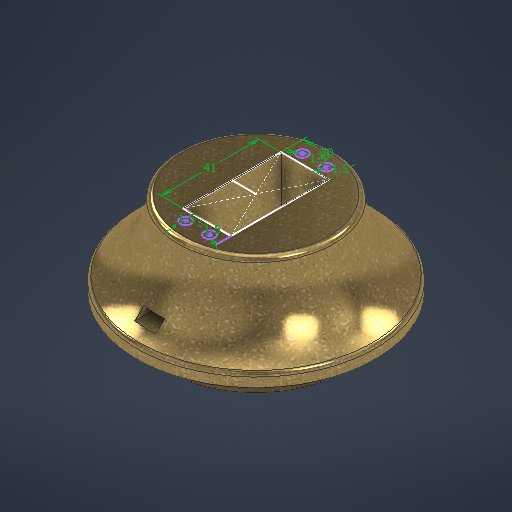
# Autodesk Inventor part: Pieza3
Saved by Autodesk Inventor 2026.1 (Build 301233020, 233B)
## iProperties
Created: 2026-05-16
Part Number: Pieza3
Material: Genérico
Document SubType Name: Modeling
Designer: USUARIO
Density: 1 g/cm^3
Appearance: Valor por defecto
Author: USUARIO
Autodesk Inventor part; units mm, degrees
ref_plane "YZ Plane" through (0, 0, 0) normal (1, 0, 0) x (0, 1, 0)
ref_plane "XZ Plane" through (0, 0, 0) normal (0, 1, 0) x (-1, 0, 0)
ref_plane "XY Plane" through (0, 0, 0) normal (0, 0, 1) x (1, 0, 0)
sketch "Boceto1" plane through (0, 0, 0) normal (1, 0, 0) x (0, 1, 0)
  line L0 (0, 0) -> (0, 32.5)
  line L1 (0, 0) -> (32.5, 0) construction
  line L2 (0, 0) -> (-35, 0)
  line L3 (0, 0) -> (35, 0) construction
  line L4 (-35, 0) -> (-35, 50)
  line L5 (-35, 0) -> (15, 0) construction
  line L6 (-35, 50) -> (-30, 50)
  line L7 (-35, 50) -> (-30, 50) construction
  arc A0 (-30, 50) -> (0, 32.5) centre (-0.3993, 66.2798) ccw
  dimension "d1" = 90
  dimension "d3" = 35
  dimension "d4" = 180
  dimension "d5" = 50
  dimension "d6" = 90
  dimension "d7" = 5
  dimension "d8" = 0
  constraints: 16 end point, 6 horizontal, 4 equal length, 2 point on circle, 2 vertical, 1 centre point
  measures "d1" angle of L1 L0
  measures "d3" distance of L0.start L2.end
  measures "d4" angle of L2 L3
  measures "d5" distance of L2.end L4.end
  measures "d6" angle of L5 L4
  measures "d7" distance of L4.end L6.end
  measures "d8" distance between parallel lines of L6 L7
revolve "Revolución1" add sketch "Boceto1" angle 360 about axis through (0, 0, 0) along (0, -1, 0)
fillet "Empalme1" radius 2 2 edges at (0, 0, -32.5) (0, -30, -50)
sketch "Boceto2" plane through (0, 0, 0) normal (0, 1, 0) x (1, 0, 0)
  line L0 (10, -20.5) -> (-10, -20.5)
  line L1 (-10, -20.5) -> (-10, 20.5)
  line L2 (-10, 20.5) -> (10, 20.5)
  line L3 (10, 20.5) -> (10, -20.5)
  line L4 (10, -20.5) -> (-10, 20.5) construction
  line L5 (-10, -20.5) -> (10, 20.5) construction
  line L6 (10, -20.5) -> (-10, -20.5)
  line L7 (10, -27) -> (10, -20.5)
  line L8 (10, -20.5) -> (-10, -20.5)
  line L9 (10, -23.5) -> (10, -20.5)
  line L10 (-10, -20.5) -> (-6, -20.5) construction
  circle A0 centre (-5, -24.5) radius 2.2
  circle A1 centre (5, -24.5) radius 2.2
  line L11 (0, 0) -> (-10, 0)
  circle A2 centre (-5, 24.5) radius 2.2
  circle A3 centre (5, 24.5) radius 2.2
  circle A4 centre (-5, 24.5) radius 0.75
  circle A5 centre (5, 24.5) radius 0.75
  circle A6 centre (-5, -24.5) radius 0.75
  circle A7 centre (5, -24.5) radius 0.75
  dimension "d11" = 20
  dimension "d12" = 41
  dimension "d34" = 1.5
  dimension "d35" = 1.5
  dimension "d36" = 1.5
  dimension "d37" = 1.5
  constraints: 24 end point, 8 centre point, 4 coincident, 4 horizontal, 3 midpoint, 2 parallel, 2 symmetric about line, 1 perpendicular, 2 other
  measures "d11" distance of L1.end L2.end
  measures "d12" distance of L0.end L1.end
  measures "d34" diameter of A4
  measures "d35" diameter of A5
  measures "d36" diameter of A6
  measures "d37" diameter of A7
extrude "Extrusión1" cut sketch "Boceto2" against normal blind 8 contours A0 | A1 | A2 | A3 | A4 | A5 | A6 | A7
extrude "Extrusión2" cut sketch "Boceto2" against normal blind 30 contours L0 L1 L2 L3
sketch "Boceto3" plane through (0, -35, 0) normal (0, -1, 0) x (1, 0, 0)
  circle A0 centre (0, 0) radius 38.5
  line L0 (38.5, 5) -> (5, 5)
  line L1 (-5, 5) -> (-38.5, 5)
  line L2 (5, 38.5) -> (5, 5)
  line L3 (5, -5) -> (5, -38.5)
  line L4 (38.5, -5) -> (5, -5)
  line L5 (-5, -5) -> (-38.5, -5)
  line L6 (-5, 38.5) -> (-5, 5)
  line L7 (-5, -5) -> (-5, -38.5)
  point P0 (38.1739, -5)
  point P1 (5, -38.1739)
  point P2 (-5, -38.1739)
  point P3 (-38.1739, -5)
  point P4 (-5, 38.1739)
  point P5 (-38.1739, 5)
  point P6 (5, 38.1739)
  point P7 (38.1739, 5)
  constraints: 16 end point, 1 centre point, 1 coincident
extrude "Extrusión3" add sketch "Boceto3" along normal blind 10 contours L0 L2 A0 | A0 L3 L4 | L6 L1 A0 | A0 L5 L7
extrude "Extrusión4" add sketch "Boceto2" against normal blind 31.25 contours A0 | A1 | A2 | A3
sketch "Boceto4" plane through (0, -35, 0) normal (0, -1, 0) x (1, 0, 0)
  line L0 (0, 0) -> (0, -39.1939)
  line L1 (0, -39.1939) -> (0, 39.081)
  line L2 (0, 0) -> (40.6258, 0)
  line L3 (40.6258, 0) -> (-47.6063, 0)
  line L4 (5, 5) -> (38.1739, 5) projected
  line L5 (-5, 5) -> (5, 5)
  line L6 (-10, -57.3754) -> (10, -57.3754)
  line L7 (10, -57.3754) -> (10, 57.3754)
  line L8 (10, 57.3754) -> (-10, 57.3754)
  line L9 (-10, 57.3754) -> (-10, -57.3754)
  line L10 (-10, -57.3754) -> (10, 57.3754) construction
  line L11 (10, -57.3754) -> (-10, 57.3754) construction
  line L12 (-59.832, 10) -> (59.832, 10)
  line L13 (59.832, 10) -> (59.832, -10)
  line L14 (59.832, -10) -> (-59.832, -10)
  line L15 (-59.832, -10) -> (-59.832, 10)
  line L16 (-59.832, 10) -> (59.832, -10) construction
  line L17 (59.832, 10) -> (-59.832, -10) construction
  point P0 (-10, -10)
  point P1 (10, -10)
  point P2 (10, 10)
  point P3 (-10, 10)
  dimension "d40" = 20
  dimension "d41" = 20
  constraints: 34 end point, 4 horizontal, 4 midpoint, 4 parallel, 2 perpendicular, 2 point on line, 1 vertical
  measures "d40" distance of L8.end L7.end
  measures "d41" distance of L12.end L13.end
extrude "Extrusión5" cut sketch "Boceto4" along normal blind 100.25
sketch "Boceto5" plane through (10, 0, 20.5) normal (0, 0, -1) x (-1, 0, 0)
  line L0 (7.039, -26.7842) -> (16.1468, -26.7842)
  line L1 (16.1468, -26.7842) -> (16.1468, -23.156)
  line L2 (16.1468, -23.156) -> (7.039, -23.156)
  line L3 (7.039, -23.156) -> (7.039, -26.7842)
  point P0 (10, 0)
  constraints: 8 end point, 2 parallel, 1 horizontal, 1 perpendicular
extrude "Extrusión6" cut sketch "Boceto5" against normal blind 100.25
